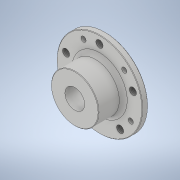
# Autodesk Inventor part: Rear_Wheel_Hub
Saved by Autodesk Inventor 2021 (Build 250183000, 183)
## iProperties
Created: 2020-10-11
Part Number: Rear_Wheel_Hub
Material: Generic
Document SubType Name: Modeling
Designer: PhotonUser
Density: 1 g/cm^3
Appearance: Default
Author: PhotonUser
Autodesk Inventor part; units mm, degrees
ref_plane "YZ Plane" through (0, 0, 0) normal (1, 0, 0) x (0, 1, 0)
ref_plane "XZ Plane" through (0, 0, 0) normal (0, 1, 0) x (-1, 0, 0)
ref_plane "XY Plane" through (0, 0, 0) normal (0, 0, 1) x (1, 0, 0)
sketch "Sketch1" plane through (0, 0, 0) normal (1, 0, 0) x (0, 1, 0)
  line L0 (0, 0) -> (38.1, 0)
  line L1 (38.1, 0) -> (38.1, -39.624)
  line L2 (38.1, -39.624) -> (68.58, -39.624)
  line L3 (68.58, -39.624) -> (68.58, -48.768)
  line L4 (68.58, -48.768) -> (32.512, -48.768)
  line L5 (32.512, -48.768) -> (32.512, -53.848)
  line L6 (32.512, -53.848) -> (28.448, -53.848)
  line L7 (28.448, -53.848) -> (28.448, -67.056)
  line L8 (28.448, -67.056) -> (0, -67.056)
  line L9 (0, -67.056) -> (0, 0)
  dimension "d0" = 38.1
  dimension "d1" = 39.624
  dimension "d2" = 30.48
  dimension "d3" = 9.144
  dimension "d4" = 36.068
  dimension "d5" = 5.08
  dimension "d6" = 4.064
  dimension "d7" = 13.208
  constraints: 20 end point, 8 perpendicular, 2 horizontal
  measures "d0" distance of L0.start L0.end
  measures "d1" distance of L0.end L1.end
  measures "d2" distance of L1.end L2.end
  measures "d3" distance of L2.end L3.end
  measures "d4" distance of L3.end L4.end
  measures "d5" distance of L4.end L5.end
  measures "d6" distance of L5.end L6.end
  measures "d7" distance of L6.end L7.end
revolve "Revolution1" add sketch "Sketch1" angle 360 about axis through (0, 0, -67.056) along (0, 0, 1)
sketch "Sketch2" plane through (0, 0, -67.056) normal (0, 0, -1) x (-1, 0, 0)
  circle A0 centre (0, 0) radius 25.4
  dimension "d9" = 50.8
  constraints: 1 centre point, 1 coincident
  measures "d9" diameter of A0
extrude "Extrusion1" cut sketch "Sketch2" against normal up to surface (18.288 mm away)
sketch "Sketch3" plane through (0, 0, -48.768) normal (0, 0, -1) x (-1, 0, 0)
  circle A0 centre (0, 0) radius 15.875
  dimension "d12" = 31.75
  constraints: 1 centre point, 1 coincident
  measures "d12" diameter of A0
extrude "Extrusion2" cut sketch "Sketch3" against normal up to surface (48.768 mm away)
fillet "Fillet1" radius 1.905 2 edges at (0, -28.448, -53.848) (0, -32.512, -48.768)
chamfer "Chamfer1" distance 0.762 angle 45 5 edges at (0, -68.58, -48.768) (0, -68.58, -39.624) (0, -38.1, 0) (0, -32.512, -53.848) (0, -28.448, -67.056)
fillet "Fillet2" radius 6.35 1 edges at (0, -38.1, -39.624)
sketch "Sketch4" plane through (0, 0, -39.624) normal (0, 0, 1) x (1, 0, 0)
  line L0 (1.6378, 0) -> (0, 0)
  line L1 (0, 0) -> (0, 80.9396)
  circle A0 centre (0, 56.388) radius 5.7404
  circle A1 centre (0, 0) radius 68.58 projected
  line L2 (0, 68.58) -> (-43.6157, 68.58)
  circle A2 centre (53.6282, 17.4249) radius 5.7404
  circle A3 centre (33.144, -45.6189) radius 5.7404
  circle A4 centre (-33.144, -45.6189) radius 5.7404
  circle A5 centre (-53.6282, 17.4249) radius 5.7404
  line L3 (0, 0) -> (47.9546, 47.9546)
  circle A6 centre (0, 0) radius 67.818 projected
  line L4 (0, 0) -> (67.818, 0) construction
  circle A7 centre (0, 0) radius 44.45 projected
  arc A8 (53.6282, 17.4249) -> (0, 56.388) centre (0, 0) ccw
  circle A9 centre (39.8723, 39.8723) radius 2.54
  dimension "d20" = 11.4808
  dimension "d21" = 12.192
  dimension "d24" = 360
  dimension "d26" = 45
  dimension "d27" = 5.08
  constraints: 10 end point, 7 centre point, 3 horizontal, 3 point on circle, 3 point on line, 2 perpendicular, 1 coincident, 1 equal length, 1 vertical alignment, 14 other
  measures "d20" diameter of A0
  measures "d21" distance from line of A0.centre L2
  measures "d26" angle of L4 L3
  measures "d27" diameter of A9
extrude "Extrusion3" cut sketch "Sketch4" against normal up to surface (9.144 mm away) contours A0 L1 | L1 A8 A0 | A9 A8 L3 | L3 A8 A9 | L1 A0 A8 | A8 A9 L3 | L3 A9 A8 | A2 | A3 | A4 | A5
thread "Thread1" size "1/2-13 UNC" class "2B" standard "ANSI Unified Screw Threads" full length
thread "Thread2" size "1/2-13 UNC" class "2B" standard "ANSI Unified Screw Threads" full length
thread "Thread3" size "1/2-13 UNC" class "2B" standard "ANSI Unified Screw Threads" full length
thread "Thread4" size "1/2-13 UNC" class "2B" standard "ANSI Unified Screw Threads" full length
thread "Thread5" size "1/2-13 UNC" class "2B" standard "ANSI Unified Screw Threads" full length
thread "Thread6" size "12-24 UNC" class "2B" standard "ANSI Unified Screw Threads" full length
sketch "Sketch5" plane through (0, 0, -48.768) normal (0, 0, -1) x (-1, 0, 0)
  circle A0 centre (0, 0) radius 44.45
  constraints: 1 centre point, 1 coincident
extrude "Extrusion4" cut sketch "Sketch5" along normal up to surface (18.288 mm away)
sketch "Sketch6" plane through (0, 0, -39.624) normal (0, 0, 1) x (1, 0, 0)
  circle A0 centre (0, 56.388) radius 5.7404 projected
  circle A1 centre (0, 0) radius 56.388
  circle A2 centre (39.8723, 39.8723) radius 2.54 projected
  circle A3 centre (39.8723, 39.8723) radius 4.1275
  circle A4 centre (-25.5996, 50.2421) radius 4.1275
  circle A5 centre (-55.6938, -8.821) radius 4.1275
  circle A6 centre (-8.821, -55.6938) radius 4.1275
  circle A7 centre (50.2421, -25.5996) radius 4.1275
  point P0 (0, 0)
  dimension "d44" = 8.255
  dimension "d47" = 360
  constraints: 5 centre point, 2 coincident, 1 vertical alignment, 13 other
  measures "d44" diameter of A3
extrude "Extrusion5" cut sketch "Sketch6" against normal blind 25.4 contours A4 A1 | A1 A4 | A3 A1 A2 | A1 A2 A3 | A5 A1 | A1 A5 | A7 A1 | A1 A7 | A6 A1 | A1 A6
equation "\"d28\" = d27"
body "Solid1"
